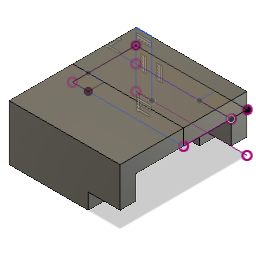
_gsdhjbx.247e5830-465d-4676-a286-db0e28371476 - Copy (Autodesk Fusion 360 design; units mm, degrees)
Autodesk Fusion 360 part; units mm, degrees
sketch "Sketch1" plane through (0, 0, 0) normal (0, 1, 0) x (1, 0, 0)
  line L0 (0, 0) -> (70, 0)
  line L1 (70, 0) -> (70, -40)
  line L2 (70, -40) -> (0, -40)
  line L3 (0, -40) -> (0, 0)
extrude "Extrude1" add sketch "Sketch1" along normal blind 10 makes body 1
sketch "Sketch2" plane through (0, 0, 0) normal (0, 1, 0) x (1, 0, 0)
  line L0 (0, 0) -> (70, 0)
  line L1 (70, 0) -> (70, -10)
  line L2 (70, -10) -> (0, -10)
  line L3 (0, -10) -> (0, 0)
  line L4 (70, -40) -> (70, 0)
extrude "Extrude2" add sketch "Sketch2" against normal blind 25 bodies 1
sketch "Sketch3" plane through (0, 0, 0) normal (0, 0, 1) x (1, 0, 0)
  line L0 (10, -25) -> (0, -25)
  line L1 (0, -25) -> (0, 10)
  line L2 (0, 10) -> (10, 10)
  line L3 (10, 10) -> (10, -25)
  line L4 (0, -25) -> (70, -25)
extrude "Extrude3" cut sketch "Sketch3" along normal blind 40 bodies 1
sketch "Sketch4" plane through (0, 0, 0) normal (0, 1, 0) x (1, 0, 0)
extrude "Extrude4" add sketch "Sketch3" along normal blind 40 bodies 1
sketch "Sketch5" plane through (0, 0, 0) normal (0, 1, 0) x (1, 0, 0)
  line L0 (0, -30) -> (10, -30)
  line L1 (10, -30) -> (10, -40)
  line L2 (10, -40) -> (0, -40)
  line L3 (0, -40) -> (0, -30)
  line L4 (0, -40) -> (0, 0)
sketch "Sketch6" plane through (0, -25, 0) normal (0, -1, 0) x (1, 0, 0)
  line L0 (0, 0) -> (70, 0)
  line L1 (70, 0) -> (70, 10)
  line L2 (70, 10) -> (10, 10)
  line L3 (10, 10) -> (10, 40)
  line L4 (10, 40) -> (0, 40)
  line L5 (0, 40) -> (0, 0)
  line L6 (0, 40) -> (10, 40)
  line L7 (10, 40) -> (10, 30)
  line L8 (10, 30) -> (0, 30)
  line L9 (0, 30) -> (0, 40)
extrude "Extrude5" cut sketch "Sketch6" against normal blind 10 contours L3 L4 L5 L6 L7 L8 L9 bodies 1
sketch "Sketch7" plane through (0, 0, 0) normal (0, 1, 0) x (1, 0, 0)
  line L0 (50, -10) -> (70, -10)
  line L1 (70, -10) -> (70, 0)
  line L2 (70, 0) -> (50, 0)
  line L3 (50, 0) -> (50, -10)
  line L4 (10, -10) -> (70, -10)
sketch "Sketch8" plane through (0, -25, 0) normal (0, -1, 0) x (1, 0, 0)
  line L0 (10, 30) -> (0, 30)
  line L1 (0, 30) -> (0, 0)
  line L2 (0, 0) -> (70, 0)
  line L3 (70, 0) -> (70, 10)
  line L4 (70, 10) -> (10, 10)
  line L5 (10, 10) -> (10, 30)
  line L6 (70, 0) -> (50, 0)
  line L7 (50, 0) -> (50, 10)
  line L8 (50, 10) -> (70, 10)
  line L9 (70, 10) -> (70, 0)
extrude "Extrude6" cut sketch "Sketch8" against normal blind 10 contours L2 L3 L4 L6 L7 L8 L9 bodies 1
mirror "Mirror1" about plane through (0, 0, 40) normal (0, 0, 1) of bodies 1 makes body 2
